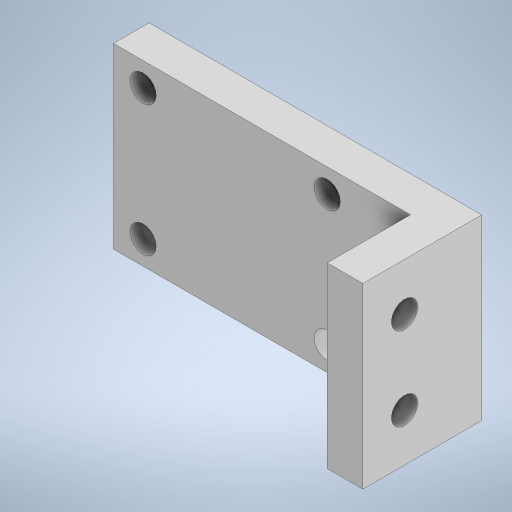
# Autodesk Inventor part: sponge_holder
Saved by Autodesk Inventor 2024.3 (Build 283343000, 343)
## iProperties
Created: 2025-06-10
Part Number: sponge_holder
Material: 一般
Document SubType Name: Modeling
Designer: hikou
Density: 1 g/cm^3
Appearance: 既定
Author: hikou
Autodesk Inventor part; units mm, degrees
ref_plane "YZ Plane" through (0, 0, 0) normal (1, 0, 0) x (0, 1, 0)
ref_plane "XZ Plane" through (0, 0, 0) normal (0, 1, 0) x (-1, 0, 0)
ref_plane "XY Plane" through (0, 0, 0) normal (0, 0, 1) x (1, 0, 0)
sketch "スケッチ1" plane through (0, 0, 0) normal (0, 0, 1) x (1, 0, 0)
  line L0 (-14, -7.5) -> (14, -7.5)
  line L1 (14, -7.5) -> (14, 7.5)
  line L2 (14, 7.5) -> (-14, 7.5)
  line L3 (-14, 7.5) -> (-14, -7.5)
  line L4 (-14, -7.5) -> (14, 7.5) construction
  line L5 (14, -7.5) -> (-14, 7.5) construction
  point P0 (0, 0)
  dimension "d0" = 28
  dimension "d1" = 15
  constraints: 12 end point, 2 midpoint, 2 parallel, 1 horizontal, 1 perpendicular
  measures "d0" distance of L1.end L2.end
  measures "d1" distance of L0.end L1.end
extrude "押し出し1" add sketch "スケッチ1" along normal mid plane 3
sketch "スケッチ2" plane through (0, 0, 1.5) normal (0, 0, 1) x (1, 0, 0)
  line L0 (14, -7.5) -> (14, 7.5) projected
  line L1 (-14, -7.5) -> (14, -7.5) projected
  line L2 (14, 7.5) -> (11, 7.5)
  line L3 (11, 7.5) -> (11, -7.5)
  line L4 (11, -7.5) -> (14, -7.5)
  line L5 (14, -7.5) -> (14, 7.5)
  point P0 (0, 0)
  dimension "d4" = 3
  constraints: 8 end point, 2 parallel, 1 horizontal, 1 perpendicular, 1 point on line
  measures "d4" distance of L4.end L3.end
extrude "押し出し2" add sketch "スケッチ2" along normal blind 7
sketch "スケッチ3" plane through (0, 0, 1.5) normal (0, 0, 1) x (1, 0, 0)
  line L0 (-14, 7.5) -> (-14, -7.5) projected
  line L1 (0, 0) -> (-2.791, 0)
  point P0 (-11.5, 5.5)
  point P1 (4, 5.5)
  point P2 (-11.5, -5.5)
  point P3 (4, -5.5)
  dimension "d7" = 15.5
  dimension "d8" = 2.5
  dimension "d9" = 5.5
  dimension "d10" = 5.5
  constraints: 2 end point, 2 symmetric about line, 1 horizontal
  measures "d7" distance of point (4, 5.5) point (-11.5, 5.5)
  measures "d8" distance from line of L0 point (-11.5, 5.5)
  measures "d9" vertical distance of L1.start point (-11.5, 5.5)
  measures "d10" vertical distance of L1.start point (4, 5.5)
hole "穴1" at (-11.5, 5.5, 1.5) at (4, 5.5, 1.5) at (-11.5, -5.5, 1.5) at (4, -5.5, 1.5) direction (0, 0, -1) diameter 2.2 end through all
sketch "スケッチ4" plane through (11, -7.5, 1.5) normal (-1, 0, 0) x (0, 0, 1)
  line L0 (0, 15) -> (7, 15) projected
  line L1 (7, 15) -> (7, 0) projected
  line L2 (0, 0) -> (7, 0) projected
  point P0 (-1.5, 7.5)
  point P1 (3.5, 11)
  point P2 (3.5, 4)
  dimension "d18" = 4
  dimension "d19" = 3.5
  dimension "d20" = 3.5
  dimension "d21" = 4
  measures "d18" distance from line of L0 point (3.5, 11)
  measures "d19" distance from line of L1 point (3.5, 11)
  measures "d20" distance from line of L1 point (3.5, 4)
  measures "d21" distance from line of L2 point (3.5, 4)
hole "穴2" at (11, 3.5, 5) at (11, -3.5, 5) direction (1, 0, 0) diameter 2.2 end through all
equation "\"d10\" = d9"
equation "\"d20\" = d19"
equation "\"d21\" = d18"
